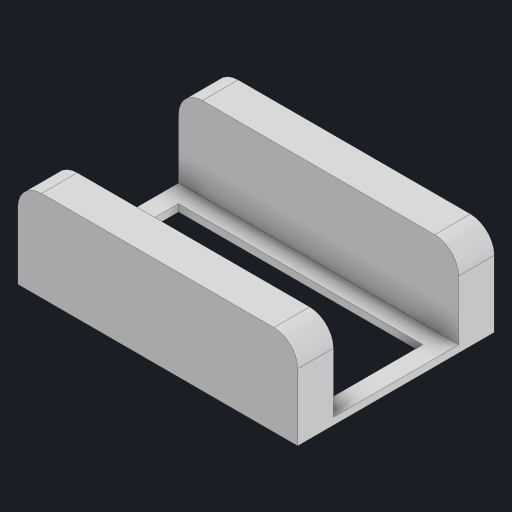
# Autodesk Inventor part: oslona_wlacznika
Saved by Autodesk Inventor 2023.4 (Build 274418000, 418)
## iProperties
Created: 2024-10-18
Part Number: oslona_wlacznika
Material: Generic
Document SubType Name: Modeling
Designer: komputer
Density: 1 g/cm^3
Appearance: Default
Author: komputer
Autodesk Inventor part; units mm, degrees
ref_plane "YZ Plane" through (0, 0, 0) normal (1, 0, 0) x (0, 1, 0)
ref_plane "XZ Plane" through (0, 0, 0) normal (0, 1, 0) x (-1, 0, 0)
ref_plane "XY Plane" through (0, 0, 0) normal (0, 0, 1) x (1, 0, 0)
sketch "Sketch1" plane through (0, 0, 0) normal (0, 1, 0) x (-1, 0, 0)
  line L0 (5.8568, 2.4857) -> (-14.6432, 2.4857)
  line L1 (-14.6432, 2.4857) -> (-14.6432, -5.0143)
  line L2 (-14.6432, -5.0143) -> (5.8568, -5.0143)
  line L3 (5.8568, -5.0143) -> (5.8568, 2.4857)
  line L4 (7.3568, 3.9857) -> (-16.1432, 3.9857)
  line L5 (-16.1432, 3.9857) -> (-16.1432, -6.5143)
  line L6 (-16.1432, -6.5143) -> (7.3568, -6.5143)
  line L7 (7.3568, -6.5143) -> (7.3568, 3.9857)
  line L8 (7.3568, 3.9857) -> (-16.1432, 3.9857)
  line L9 (-16.1432, 3.9857) -> (-16.1432, 6.9857)
  line L10 (-16.1432, 6.9857) -> (7.3568, 6.9857)
  line L11 (7.3568, 6.9857) -> (7.3568, 3.9857)
  line L12 (7.3568, -6.5143) -> (-16.1432, -6.5143)
  line L13 (-16.1432, -6.5143) -> (-16.1432, -9.5143)
  line L14 (-16.1432, -9.5143) -> (7.3568, -9.5143)
  line L15 (7.3568, -9.5143) -> (7.3568, -6.5143)
  point P0 (0, 0)
  dimension "d0" = 20.5
  dimension "d1" = 7.5
  dimension "d2" = 1.5
  dimension "d3" = 3
  dimension "d4" = 3
  constraints: 32 end point, 8 parallel, 4 perpendicular, 3 horizontal, 1 point on line, 1 vertical alignment, 3 other
  measures "d0" distance of L2.end L1.end
  measures "d1" distance of L1.end L0.end
  measures "d2" distance between parallel lines of L3 L7
  measures "d3" distance between parallel lines of L4 L10
  measures "d4" distance between parallel lines of L14 L12
extrude "Extrusion1" add sketch "Sketch1" along normal blind 0.6 contours L7 L6 L5 L4
extrude "Extrusion2" add sketch "Sketch1" along normal blind 7.6 contours L4 L9 L10 L11 | L15 L14 L13 L6
fillet "Fillet1" radius 2 4 edges at (-7.3568, 7.6, 5.4857) (16.1432, 7.6, -8.0143) (16.1432, 7.6, 5.4857) (-7.3568, 7.6, -8.0143)
body "Solid1"
